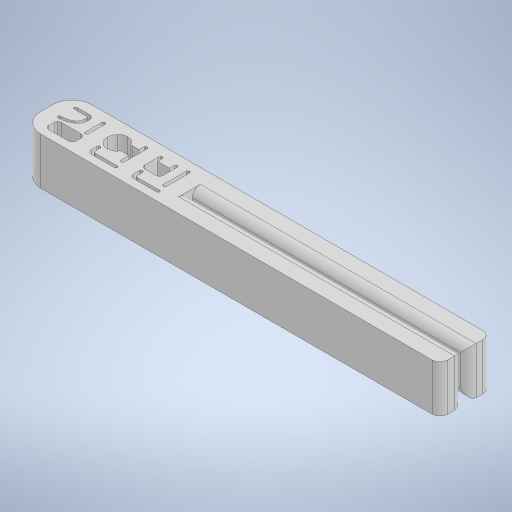
# Autodesk Inventor part: part2
Saved by Autodesk Inventor 2024 (Build 280153000, 153)
## iProperties
Created: 2023-11-09
Part Number: part2
Material: 일반
Document SubType Name: Modeling
Designer: SSAFY
Density: 1 g/cm^3
Appearance: 기본값
Author: SSAFY
Autodesk Inventor part; units mm, degrees
ref_plane "YZ Plane" through (0, 0, 0) normal (1, 0, 0) x (0, 1, 0)
ref_plane "XZ Plane" through (0, 0, 0) normal (0, 1, 0) x (-1, 0, 0)
ref_plane "XY Plane" through (0, 0, 0) normal (0, 0, 1) x (1, 0, 0)
sketch "스케치1" plane through (0, 0, 0) normal (0, 0, 1) x (1, 0, 0)
  point P0 (0, 0)
sketch "스케치2" plane through (0, 0, 0) normal (0, 1, 0) x (-1, 0, 0)
  line L0 (-38.5, 6.5) -> (38.5, 6.5)
  line L1 (38.5, 6.5) -> (38.5, -6.5)
  line L2 (38.5, -6.5) -> (-38.5, -6.5)
  line L3 (-38.5, -6.5) -> (-38.5, 6.5)
  line L4 (-38.5, 6.5) -> (38.5, -6.5) construction
  line L5 (38.5, 6.5) -> (-38.5, -6.5) construction
  line L6 (-32, 0.75) -> (32, 0.75)
  line L7 (32, 0.75) -> (32, -0.75)
  line L8 (32, -0.75) -> (-32, -0.75)
  line L9 (-32, -0.75) -> (-32, 0.75)
  line L10 (-32, 0.75) -> (32, -0.75) construction
  line L11 (32, 0.75) -> (-32, -0.75) construction
  line L12 (-32, 0.75) -> (-38.5, 0.75)
  line L13 (-38.5, 0.75) -> (-38.5, -0.75)
  line L14 (-38.5, -0.75) -> (-32, -0.75)
  line L15 (-32, -0.75) -> (-32, 0.75)
  point P0 (0, 0)
  point P1 (-32, -0.5)
  dimension "d0" = 77
  dimension "d1" = 13
  dimension "d2" = 64
  dimension "d3" = 1.5
  constraints: 32 end point, 6 parallel, 4 midpoint, 3 horizontal, 3 perpendicular, 1 point on line
  measures "d0" distance of L1.end L2.end
  measures "d1" distance of L2.end L0.start
  measures "d2" distance of L7.end L8.end
  measures "d3" distance of L8.end L6.start
extrude "돌출1" add sketch "스케치2" along normal mid plane 12 contours L0 L1 L2 L3 L14 L8 L7 L6 L12
sketch "스케치5" plane through (-38.5, -6, 6.5) normal (-1, 0, 0) x (0, 0, 1)
  line L0 (-13, 12) -> (0, 12)
  line L1 (0, 12) -> (0, 0)
  line L2 (0, 0) -> (-13, 0)
  line L3 (-13, 0) -> (-13, 12)
  point P0 (-6.5, 6)
  constraints: 8 end point, 2 parallel, 1 horizontal, 1 perpendicular
extrude "돌출3" add sketch "스케치5" along normal blind 30
sketch "스케치7" plane through (0, 6, 0) normal (0, 1, 0) x (1, 0, 0)
  line L0 (-67.5541, 5.3583) -> (-32.9181, 5.3583) construction
  line L1 (-32.9181, 5.3583) -> (-32.9181, -5.6155) construction
  line L2 (-32.9181, -5.6155) -> (-67.5541, -5.6155) construction
  line L3 (-67.5541, -5.6155) -> (-67.5541, 5.3583) construction
  line L4 (-58.4922, -1.2761) -> (-63.4387, -1.2761)
  spline S0 degree 2 poles (-63.4387, -1.2761) (-63.8795, -1.2761) (-64.1388, -1.5289) knots 0 0 0 1 1 1
  spline S1 degree 2 poles (-64.1388, -1.5289) (-64.4046, -1.7818) (-64.4046, -2.1578) knots 0 0 0 1 1 1
  line L5 (-64.4046, -2.1578) -> (-64.4046, -3.5451)
  spline S2 degree 2 poles (-64.4046, -3.5451) (-64.4046, -4.0119) (-64.1518, -4.2583) knots 0 0 0 1 1 1
  spline S3 degree 2 poles (-64.1518, -4.2583) (-63.8795, -4.5176) (-63.3025, -4.5176) knots 0 0 0 1 1 1
  line L6 (-63.3025, -4.5176) -> (-58.4468, -4.5176)
  spline S4 degree 2 poles (-58.4468, -4.5176) (-57.9865, -4.5176) (-57.6753, -4.1286) knots 0 0 0 1 1 1
  spline S5 degree 2 poles (-57.6753, -4.1286) (-57.4225, -4.0508) (-57.4225, -3.597) knots 0 0 0 1 1 1
  line L7 (-57.4225, -3.597) -> (-57.4225, -2.1189)
  spline S6 degree 2 poles (-57.4225, -2.1189) (-57.4225, -1.7364) (-57.6753, -1.5289) knots 0 0 0 1 1 1
  spline S7 degree 2 poles (-57.6753, -1.5289) (-58.0124, -1.2761) (-58.4922, -1.2761) knots 0 0 0 1 1 1
  line L8 (-58.2782, -2.2745) -> (-58.2782, -3.5322)
  spline S8 degree 2 poles (-58.2782, -3.5322) (-58.2782, -3.6618) (-58.3301, -3.7007) knots 0 0 0 1 1 1
  spline S9 degree 2 poles (-58.3301, -3.7007) (-58.4273, -3.7656) (-58.6283, -3.7656) knots 0 0 0 1 1 1
  line L9 (-58.6283, -3.7656) -> (-63.1858, -3.7656)
  spline S10 degree 2 poles (-63.1858, -3.7656) (-63.4192, -3.7656) (-63.497, -3.7007) knots 0 0 0 1 1 1
  spline S11 degree 2 poles (-63.497, -3.7007) (-63.5489, -3.6553) (-63.5489, -3.4868) knots 0 0 0 1 1 1
  line L10 (-63.5489, -3.4868) -> (-63.5489, -2.3004)
  spline S12 degree 2 poles (-63.5489, -2.3004) (-63.5489, -2.1448) (-63.4841, -2.08) knots 0 0 0 1 1 1
  spline S13 degree 2 poles (-63.4841, -2.08) (-63.4257, -2.0281) (-63.2183, -2.0281) knots 0 0 0 1 1 1
  line L11 (-63.2183, -2.0281) -> (-58.6413, -2.0281)
  spline S14 degree 2 poles (-58.6413, -2.0281) (-58.4273, -2.0281) (-58.3301, -2.0929) knots 0 0 0 1 1 1
  spline S15 degree 2 poles (-58.3301, -2.0929) (-58.2782, -2.1318) (-58.2782, -2.2745) knots 0 0 0 1 1 1
  line L12 (-61.5262, 4.0075) -> (-64.7482, 4.0075)
  spline S16 degree 2 poles (-64.7482, 4.0075) (-65.1567, 4.0075) (-65.1437, 3.638) knots 0 0 0 1 1 1
  spline S17 degree 2 poles (-65.1437, 3.638) (-65.1437, 3.2555) (-64.7418, 3.2555) knots 0 0 0 1 1 1
  line L13 (-64.7418, 3.2555) -> (-61.591, 3.2555)
  spline S18 degree 2 poles (-61.591, 3.2555) (-61.4095, 3.2555) (-61.3252, 3.1842) knots 0 0 0 1 1 1
  spline S19 degree 2 poles (-61.3252, 3.1842) (-61.215, 3.0999) (-61.215, 2.9314) knots 0 0 0 1 1 1
  line L14 (-61.215, 2.9314) -> (-61.215, 2.4711)
  spline S20 degree 2 poles (-61.215, 2.4711) (-61.215, 1.3366) (-62.0319, 0.7272) knots 0 0 0 1 1 1
  spline S21 degree 2 poles (-62.0319, 0.7272) (-63.0886, 0.0789) (-64.8455, 0.0075) knots 0 0 0 1 1 1
  spline S22 degree 2 poles (-64.8455, 0.0075) (-65.0918, 0.0075) (-65.215, -0.1156) knots 0 0 0 1 1 1
  spline S23 degree 2 poles (-65.215, -0.1156) (-65.3187, -0.2258) (-65.3187, -0.3814) knots 0 0 0 1 1 1
  spline S24 degree 2 poles (-65.3187, -0.3814) (-65.3187, -0.5435) (-65.1826, -0.6472) knots 0 0 0 1 1 1
  spline S25 degree 2 poles (-65.1826, -0.6472) (-65.0594, -0.7445) (-64.8585, -0.7445) knots 0 0 0 1 1 1
  spline S26 degree 2 poles (-64.8585, -0.7445) (-62.7515, -0.6472) (-61.5781, 0.202) knots 0 0 0 1 1 1
  spline S27 degree 2 poles (-61.5781, 0.202) (-60.3917, 1.0578) (-60.3917, 2.4646) knots 0 0 0 1 1 1
  line L15 (-60.3917, 2.4646) -> (-60.3917, 3.0221)
  spline S28 degree 2 poles (-60.3917, 3.0221) (-60.3917, 3.463) (-60.7353, 3.7482) knots 0 0 0 1 1 1
  spline S29 degree 2 poles (-60.7353, 3.7482) (-61.04, 4.0075) (-61.5262, 4.0075) knots 0 0 0 1 1 1
  line L16 (-57.4225, -0.3296) -> (-57.4225, 3.8714)
  spline S30 degree 2 poles (-57.4225, 3.8714) (-57.4225, 4.0594) (-57.5716, 4.1631) knots 0 0 0 1 1 1
  spline S31 degree 2 poles (-57.5716, 4.1631) (-57.6818, 4.2604) (-57.8504, 4.2604) knots 0 0 0 1 1 1
  spline S32 degree 2 poles (-57.8504, 4.2604) (-58.0319, 4.2604) (-58.1486, 4.1631) knots 0 0 0 1 1 1
  spline S33 degree 2 poles (-58.1486, 4.1631) (-58.2782, 4.04) (-58.2782, 3.8649) knots 0 0 0 1 1 1
  line L17 (-58.2782, 3.8649) -> (-58.2782, -0.3296)
  spline S34 degree 2 poles (-58.2782, -0.3296) (-58.2782, -0.5241) (-58.1551, -0.6472) knots 0 0 0 1 1 1
  spline S35 degree 2 poles (-58.1551, -0.6472) (-58.0384, -0.7639) (-57.8504, -0.7639) knots 0 0 0 1 1 1
  spline S36 degree 2 poles (-57.8504, -0.7639) (-57.6753, -0.7639) (-57.5457, -0.6343) knots 0 0 0 1 1 1
  spline S37 degree 2 poles (-57.5457, -0.6343) (-57.4225, -0.5241) (-57.4225, -0.3296) knots 0 0 0 1 1 1
  spline S38 degree 2 poles (-51.7628, 3.9881) (-52.9622, 3.9881) (-53.6688, 3.1583) knots 0 0 0 1 1 1
  spline S39 degree 2 poles (-53.6688, 3.1583) (-54.2977, 2.4257) (-54.2977, 1.356) knots 0 0 0 1 1 1
  spline S40 degree 2 poles (-54.2977, 1.356) (-54.2977, 0.2928) (-53.6948, -0.3425) knots 0 0 0 1 1 1
  spline S41 degree 2 poles (-53.6948, -0.3425) (-52.9622, -1.2826) (-51.7628, -1.2826) knots 0 0 0 1 1 1
  spline S42 degree 2 poles (-51.7628, -1.2826) (-50.5829, -1.2826) (-49.8893, -0.4527) knots 0 0 0 1 1 1
  spline S43 degree 2 poles (-49.8893, -0.4527) (-49.2604, 0.2863) (-49.2604, 1.356) knots 0 0 0 1 1 1
  spline S44 degree 2 poles (-49.2604, 1.356) (-49.2604, 2.4257) (-49.8893, 3.1583) knots 0 0 0 1 1 1
  spline S45 degree 2 poles (-49.8893, 3.1583) (-50.5829, 3.9881) (-51.7628, 3.9881) knots 0 0 0 1 1 1
  spline S46 degree 2 poles (-51.7628, 3.2361) (-50.9654, 3.2361) (-50.5181, 2.6656) knots 0 0 0 1 1 1
  spline S47 degree 2 poles (-50.5181, 2.6656) (-50.0902, 2.134) (-50.0902, 1.356) knots 0 0 0 1 1 1
  spline S48 degree 2 poles (-50.0902, 1.356) (-50.0902, 0.5716) (-50.5246, 0.0335) knots 0 0 0 1 1 1
  spline S49 degree 2 poles (-50.5246, 0.0335) (-50.9654, -0.5305) (-51.7628, -0.5305) knots 0 0 0 1 1 1
  spline S50 degree 2 poles (-51.7628, -0.5305) (-52.5797, -0.5305) (-53.0335, 0.0529) knots 0 0 0 1 1 1
  spline S51 degree 2 poles (-53.0335, 0.0529) (-53.4419, 0.5651) (-53.4419, 1.356) knots 0 0 0 1 1 1
  spline S52 degree 2 poles (-53.4419, 1.356) (-53.4419, 2.1404) (-53.0335, 2.6591) knots 0 0 0 1 1 1
  spline S53 degree 2 poles (-53.0335, 2.6591) (-52.5732, 3.2361) (-51.7628, 3.2361) knots 0 0 0 1 1 1
  line L18 (-46.6283, -1.9438) -> (-46.6283, 3.8714)
  spline S54 degree 2 poles (-46.6283, 3.8714) (-46.6283, 4.0594) (-46.7709, 4.1567) knots 0 0 0 1 1 1
  spline S55 degree 2 poles (-46.7709, 4.1567) (-46.8876, 4.2604) (-47.0562, 4.2604) knots 0 0 0 1 1 1
  spline S56 degree 2 poles (-47.0562, 4.2604) (-47.2377, 4.2604) (-47.3544, 4.1631) knots 0 0 0 1 1 1
  spline S57 degree 2 poles (-47.3544, 4.1631) (-47.4841, 4.0464) (-47.4841, 3.8649) knots 0 0 0 1 1 1
  line L19 (-47.4841, 3.8649) -> (-47.4841, 2.6202)
  line L20 (-47.4841, 2.6202) -> (-49.1696, 2.6202)
  spline S58 degree 2 poles (-49.1696, 2.6202) (-49.3771, 2.6202) (-49.4938, 2.5165) knots 0 0 0 1 1 1
  spline S59 degree 2 poles (-49.4938, 2.5165) (-49.5975, 2.3998) (-49.5975, 2.2377) knots 0 0 0 1 1 1
  spline S60 degree 2 poles (-49.5975, 2.2377) (-49.5846, 2.0951) (-49.4743, 1.9849) knots 0 0 0 1 1 1
  spline S61 degree 2 poles (-49.4743, 1.9849) (-49.3252, 1.8682) (-49.1178, 1.8682) knots 0 0 0 1 1 1
  line L21 (-49.1178, 1.8682) -> (-47.4841, 1.8682)
  line L22 (-47.4841, 1.8682) -> (-47.4841, 0.7012)
  line L23 (-47.4841, 0.7012) -> (-49.1502, 0.7012)
  spline S62 degree 2 poles (-49.1502, 0.7012) (-49.3447, 0.7012) (-49.4808, 0.5975) knots 0 0 0 1 1 1
  spline S63 degree 2 poles (-49.4808, 0.5975) (-49.5846, 0.4938) (-49.5846, 0.3382) knots 0 0 0 1 1 1
  spline S64 degree 2 poles (-49.5846, 0.3382) (-49.5846, 0.1761) (-49.4614, 0.0724) knots 0 0 0 1 1 1
  spline S65 degree 2 poles (-49.4614, 0.0724) (-49.3382, -0.0378) (-49.1372, -0.0378) knots 0 0 0 1 1 1
  line L24 (-49.1372, -0.0378) -> (-47.4841, -0.0378)
  line L25 (-47.4841, -0.0378) -> (-47.4841, -1.9438)
  spline S66 degree 2 poles (-47.4841, -1.9438) (-47.4841, -2.1513) (-47.3609, -2.2745) knots 0 0 0 1 1 1
  spline S67 degree 2 poles (-47.3609, -2.2745) (-47.2442, -2.3912) (-47.0562, -2.3912) knots 0 0 0 1 1 1
  spline S68 degree 2 poles (-47.0562, -2.3912) (-46.8811, -2.3912) (-46.7515, -2.2615) knots 0 0 0 1 1 1
  spline S69 degree 2 poles (-46.7515, -2.2615) (-46.6283, -2.1513) (-46.6283, -1.9438) knots 0 0 0 1 1 1
  spline S70 degree 2 poles (-52.7677, -2.067) (-52.7677, -1.8531) (-52.8909, -1.7429) knots 0 0 0 1 1 1
  spline S71 degree 2 poles (-52.8909, -1.7429) (-53.0205, -1.6132) (-53.1956, -1.6132) knots 0 0 0 1 1 1
  spline S72 degree 2 poles (-53.1956, -1.6132) (-53.3836, -1.6132) (-53.5003, -1.7299) knots 0 0 0 1 1 1
  spline S73 degree 2 poles (-53.5003, -1.7299) (-53.6234, -1.8531) (-53.6234, -2.067) knots 0 0 0 1 1 1
  line L26 (-53.6234, -2.067) -> (-53.6234, -3.4673)
  spline S74 degree 2 poles (-53.6234, -3.4673) (-53.6234, -3.986) (-53.2799, -4.2712) knots 0 0 0 1 1 1
  spline S75 degree 2 poles (-53.2799, -4.2712) (-52.9881, -4.5176) (-52.4695, -4.5176) knots 0 0 0 1 1 1
  line L27 (-52.4695, -4.5176) -> (-46.6867, -4.5176)
  spline S76 degree 2 poles (-46.6867, -4.5176) (-46.3106, -4.5176) (-46.3106, -4.1351) knots 0 0 0 1 1 1
  spline S77 degree 2 poles (-46.3106, -4.1351) (-46.3106, -3.7656) (-46.6867, -3.7656) knots 0 0 0 1 1 1
  line L28 (-46.6867, -3.7656) -> (-52.3593, -3.7656)
  spline S78 degree 2 poles (-52.3593, -3.7656) (-52.6251, -3.7656) (-52.6834, -3.7137) knots 0 0 0 1 1 1
  spline S79 degree 2 poles (-52.6834, -3.7137) (-52.7677, -3.6294) (-52.7677, -3.3831) knots 0 0 0 1 1 1
  line L29 (-52.7677, -3.3831) -> (-52.7677, -2.067)
  line L30 (-39.5165, 3.5991) -> (-39.5165, 2.3868)
  line L31 (-39.5165, 2.3868) -> (-42.5311, 2.3868)
  line L32 (-42.5311, 2.3868) -> (-42.5311, 3.5473)
  spline S80 degree 2 poles (-42.5311, 3.5473) (-42.5311, 3.7612) (-42.6542, 3.8714) knots 0 0 0 1 1 1
  spline S81 degree 2 poles (-42.6542, 3.8714) (-42.7839, 4.0011) (-42.9589, 4.0011) knots 0 0 0 1 1 1
  spline S82 degree 2 poles (-42.9589, 4.0011) (-43.134, 4.0011) (-43.2377, 3.8844) knots 0 0 0 1 1 1
  spline S83 degree 2 poles (-43.2377, 3.8844) (-43.3739, 3.7482) (-43.3739, 3.5408) knots 0 0 0 1 1 1
  line L33 (-43.3739, 3.5408) -> (-43.3739, -0.0443)
  spline S84 degree 2 poles (-43.3739, -0.0443) (-43.3739, -0.4852) (-43.1081, -0.7186) knots 0 0 0 1 1 1
  spline S85 degree 2 poles (-43.1081, -0.7186) (-42.8098, -0.9649) (-42.3755, -0.9649) knots 0 0 0 1 1 1
  line L34 (-42.3755, -0.9649) -> (-39.7304, -0.9649)
  spline S86 degree 2 poles (-39.7304, -0.9649) (-39.2766, -0.9649) (-38.9978, -0.7121) knots 0 0 0 1 1 1
  spline S87 degree 2 poles (-38.9978, -0.7121) (-38.6931, -0.4527) (-38.6931, -0.0443) knots 0 0 0 1 1 1
  line L35 (-38.6931, -0.0443) -> (-38.6931, 3.5926)
  spline S88 degree 2 poles (-38.6931, 3.5926) (-38.6931, 4.0011) (-39.1081, 4.0011) knots 0 0 0 1 1 1
  spline S89 degree 2 poles (-39.1081, 4.0011) (-39.5165, 4.0011) (-39.5165, 3.5991) knots 0 0 0 1 1 1
  spline S90 degree 2 poles (-41.9735, -2.067) (-41.9735, -1.8531) (-42.0967, -1.7429) knots 0 0 0 1 1 1
  spline S91 degree 2 poles (-42.0967, -1.7429) (-42.2264, -1.6132) (-42.4014, -1.6132) knots 0 0 0 1 1 1
  spline S92 degree 2 poles (-42.4014, -1.6132) (-42.5894, -1.6132) (-42.7061, -1.7299) knots 0 0 0 1 1 1
  spline S93 degree 2 poles (-42.7061, -1.7299) (-42.8293, -1.8531) (-42.8293, -2.067) knots 0 0 0 1 1 1
  line L36 (-42.8293, -2.067) -> (-42.8293, -3.4673)
  spline S94 degree 2 poles (-42.8293, -3.4673) (-42.8293, -3.986) (-42.4857, -4.2712) knots 0 0 0 1 1 1
  spline S95 degree 2 poles (-42.4857, -4.2712) (-42.194, -4.5176) (-41.6753, -4.5176) knots 0 0 0 1 1 1
  line L37 (-41.6753, -4.5176) -> (-35.8925, -4.5176)
  spline S96 degree 2 poles (-35.8925, -4.5176) (-35.5165, -4.5176) (-35.5165, -4.1351) knots 0 0 0 1 1 1
  spline S97 degree 2 poles (-35.5165, -4.1351) (-35.5165, -3.7656) (-35.8925, -3.7656) knots 0 0 0 1 1 1
  line L38 (-35.8925, -3.7656) -> (-41.5651, -3.7656)
  spline S98 degree 2 poles (-41.5651, -3.7656) (-41.8309, -3.7656) (-41.8893, -3.7137) knots 0 0 0 1 1 1
  spline S99 degree 2 poles (-41.8893, -3.7137) (-41.9735, -3.6294) (-41.9735, -3.3831) knots 0 0 0 1 1 1
  line L39 (-41.9735, -3.3831) -> (-41.9735, -2.067)
  line L40 (-35.8341, -1.9438) -> (-35.8341, 3.8714)
  spline S100 degree 2 poles (-35.8341, 3.8714) (-35.8341, 4.0594) (-35.9768, 4.1567) knots 0 0 0 1 1 1
  spline S101 degree 2 poles (-35.9768, 4.1567) (-36.0935, 4.2604) (-36.262, 4.2604) knots 0 0 0 1 1 1
  spline S102 degree 2 poles (-36.262, 4.2604) (-36.4435, 4.2604) (-36.5602, 4.1631) knots 0 0 0 1 1 1
  spline S103 degree 2 poles (-36.5602, 4.1631) (-36.6899, 4.04) (-36.6899, 3.8649) knots 0 0 0 1 1 1
  line L41 (-36.6899, 3.8649) -> (-36.6899, -1.9438)
  spline S104 degree 2 poles (-36.6899, -1.9438) (-36.6899, -2.1513) (-36.5667, -2.2745) knots 0 0 0 1 1 1
  spline S105 degree 2 poles (-36.5667, -2.2745) (-36.45, -2.3912) (-36.262, -2.3912) knots 0 0 0 1 1 1
  spline S106 degree 2 poles (-36.262, -2.3912) (-36.087, -2.3912) (-35.9573, -2.2615) knots 0 0 0 1 1 1
  spline S107 degree 2 poles (-35.9573, -2.2615) (-35.8341, -2.1513) (-35.8341, -1.9438) knots 0 0 0 1 1 1
  line L42 (-39.5165, 1.6348) -> (-39.5165, 0.0853)
  spline S108 degree 2 poles (-39.5165, 0.0853) (-39.5165, -0.0767) (-39.6137, -0.1416) knots 0 0 0 1 1 1
  spline S109 degree 2 poles (-39.6137, -0.1416) (-39.698, -0.2129) (-39.9119, -0.2129) knots 0 0 0 1 1 1
  line L43 (-39.9119, -0.2129) -> (-42.2069, -0.2129)
  spline S110 degree 2 poles (-42.2069, -0.2129) (-42.4079, -0.2129) (-42.4598, -0.161) knots 0 0 0 1 1 1
  spline S111 degree 2 poles (-42.4598, -0.161) (-42.5311, -0.1027) (-42.5311, 0.0853) knots 0 0 0 1 1 1
  line L44 (-42.5311, 0.0853) -> (-42.5311, 1.6348)
  line L45 (-42.5311, 1.6348) -> (-39.5165, 1.6348)
  point P0 (0, 0)
  constraints: 2 other
emboss "엠보싱3" sketch "스케치7" operation cut depth 15 direction (0, -1, 0) contours S7 S6 L7 S5 S4 L6 S3 S2 L5 S1 S0 L4 | S29 S28 L15 S27 S26 S25 S24 S23 S22 S21 S20 L14 S19 S18 L13 S17 S16 L12 | S37 S36 S35 S34 L17 S33 S32 S31 S30 L16 | S45 S44 S58 S59 S60 S61 S43 S62 S63 S64 S42 S41 S40 S39 S38 | S58 L20 L19 S57 S56 S55 S54 L18 S69 S68 S67 S66 L25 L24 S65 S64 S43 S62 L23 L22 L21 S61 S44 | S44 S61 S60 S59 S58 | S43 S64 S63 S62 | L29 S79 S78 L28 S77 S76 L27 S75 S74 L26 S73 S72 S71 S70 | S89 S88 L35 S87 S86 L34 S85 S84 L33 S83 S82 S81 S80 L32 L31 L30 | L39 S99 S98 L38 S97 S96 L37 S95 S94 L36 S93 S92 S91 S90 | S107 S106 S105 S104 L41 S103 S102 S101 S100 L40
sketch "스케치8" plane through (0, 6, 0) normal (0, 1, 0) x (1, 0, 0)
  spline S0 degree 6 poles (-63.497, -3.7007) (-63.4703, -3.723) (-63.4326, -3.7406) (-63.3844, -3.7534) (-63.3266, -3.7616) (-63.2601, -3.7656) (-63.1858, -3.7656) knots 0 0 0 0 0 0 0 1 1 1 1 1 1 1 projected
  line L0 (-63.1858, -3.7656) -> (-58.6283, -3.7656) projected
  spline S1 degree 5 poles (-58.6283, -3.7656) (-58.5502, -3.7656) (-58.4804, -3.7594) (-58.42, -3.7467) (-58.3698, -3.7272) (-58.3301, -3.7007) knots 0 0 0 0 0 0 1 1 1 1 1 1 projected
  spline S2 degree 5 poles (-58.3301, -3.7007) (-58.3092, -3.685) (-58.2935, -3.6601) (-58.2833, -3.6261) (-58.2782, -3.5832) (-58.2782, -3.5322) knots 0 0 0 0 0 0 1 1 1 1 1 1 projected
  line L1 (-58.2782, -3.5322) -> (-58.2782, -2.2745) projected
  spline S3 degree 5 poles (-58.2782, -2.2745) (-58.2782, -2.2185) (-58.2832, -2.1718) (-58.2935, -2.135) (-58.3091, -2.1087) (-58.3301, -2.0929) knots 0 0 0 0 0 0 1 1 1 1 1 1 projected
  spline S4 degree 5 poles (-58.3301, -2.0929) (-58.3699, -2.0664) (-58.4218, -2.0468) (-58.485, -2.0342) (-58.5585, -2.0281) (-58.6413, -2.0281) knots 0 0 0 0 0 0 1 1 1 1 1 1 projected
  line L2 (-58.6413, -2.0281) -> (-63.2183, -2.0281) projected
  spline S5 degree 6 poles (-63.2183, -2.0281) (-63.2847, -2.0281) (-63.3433, -2.0313) (-63.3932, -2.0379) (-63.4337, -2.0482) (-63.4641, -2.0622) (-63.4841, -2.08) knots 0 0 0 0 0 0 0 1 1 1 1 1 1 1 projected
  spline S6 degree 5 poles (-63.4841, -2.08) (-63.5103, -2.1062) (-63.5298, -2.1417) (-63.5426, -2.1862) (-63.5489, -2.2393) (-63.5489, -2.3004) knots 0 0 0 0 0 0 1 1 1 1 1 1 projected
  line L3 (-63.5489, -2.3004) -> (-63.5489, -3.4868) projected
  spline S7 degree 5 poles (-63.5489, -3.4868) (-63.5489, -3.5524) (-63.544, -3.6075) (-63.5338, -3.6511) (-63.5181, -3.6823) (-63.497, -3.7007) knots 0 0 0 0 0 0 1 1 1 1 1 1 projected
  spline S8 degree 5 poles (-51.7628, -0.5305) (-51.6946, -0.5305) (-51.6268, -0.528) (-51.5597, -0.5226) (-51.4932, -0.5143) (-51.3117, -0.4829) (-51.1986, -0.453) (-51.0897, -0.4127) (-50.9863, -0.3616) (-50.806, -0.2475) (-50.7274, -0.1872) (-50.6542, -0.1197) (-50.5866, -0.0459) (-50.5246, 0.0335) knots 0 0 0 0 0 0 0.232634 0.232634 0.232634 0.232634 0.645224 0.645224 0.645224 0.645224 1 1 1 1 1 1 projected
  spline S9 degree 6 poles (-50.5246, 0.0335) (-50.4921, 0.0738) (-50.4609, 0.115) (-50.4311, 0.1573) (-50.4027, 0.2004) (-50.3758, 0.2444) (-50.2608, 0.4477) (-50.1896, 0.6166) (-50.1381, 0.7941) (-50.1055, 0.9779) (-50.0902, 1.1658) (-50.0902, 1.356) knots 0 0 0 0 0 0 0 0.220725 0.220725 0.220725 0.220725 0.220725 1 1 1 1 1 1 1 projected
  spline S10 degree 6 poles (-50.0902, 1.356) (-50.0902, 1.5473) (-50.1058, 1.7362) (-50.1388, 1.9209) (-50.1911, 2.0991) (-50.2634, 2.2684) (-50.3786, 2.4685) (-50.404, 2.5096) (-50.4306, 2.5498) (-50.4586, 2.5893) (-50.4877, 2.6278) (-50.5181, 2.6656) knots 0 0 0 0 0 0 0 0.791229 0.791229 0.791229 0.791229 0.791229 1 1 1 1 1 1 1 projected
  spline S11 degree 5 poles (-50.5181, 2.6656) (-50.5837, 2.7492) (-50.6553, 2.8269) (-50.733, 2.8975) (-50.8165, 2.9603) (-51.0015, 3.0738) (-51.104, 3.1231) (-51.2117, 3.1619) (-51.3232, 3.1906) (-51.5012, 3.2207) (-51.5657, 3.2285) (-51.6309, 3.2336) (-51.6967, 3.2361) (-51.7628, 3.2361) knots 0 0 0 0 0 0 0.371373 0.371373 0.371373 0.371373 0.775292 0.775292 0.775292 0.775292 1 1 1 1 1 1 projected
  spline S12 degree 5 poles (-51.7628, 3.2361) (-51.8301, 3.2361) (-51.897, 3.2336) (-51.9633, 3.2285) (-52.0289, 3.2205) (-52.2101, 3.1901) (-52.3238, 3.1611) (-52.4335, 3.1218) (-52.5381, 3.0719) (-52.7273, 2.9571) (-52.8128, 2.8937) (-52.8925, 2.8222) (-52.966, 2.7437) (-53.0335, 2.6591) knots 0 0 0 0 0 0 0.224613 0.224613 0.224613 0.224613 0.628567 0.628567 0.628567 0.628567 1 1 1 1 1 1 projected
  spline S13 degree 6 poles (-53.0335, 2.6591) (-53.0501, 2.638) (-53.0663, 2.6167) (-53.0821, 2.5951) (-53.0975, 2.5732) (-53.1125, 2.551) (-53.2366, 2.3603) (-53.3232, 2.1772) (-53.3852, 1.9819) (-53.4239, 1.778) (-53.4419, 1.5685) (-53.4419, 1.356) knots 0 0 0 0 0 0 0 0.117636 0.117636 0.117636 0.117636 0.117636 1 1 1 1 1 1 1 projected
  spline S14 degree 6 poles (-53.4419, 1.356) (-53.4419, 1.2427) (-53.4369, 1.1303) (-53.4264, 1.0192) (-53.4101, 0.9098) (-53.3875, 0.8026) (-53.3314, 0.6005) (-53.2988, 0.5054) (-53.2603, 0.4129) (-53.2158, 0.3236) (-53.1656, 0.2379) (-53.0976, 0.1384) (-53.0853, 0.1209) (-53.0727, 0.1036) (-53.0599, 0.0865) (-53.0468, 0.0696) (-53.0335, 0.0529) knots 0 0 0 0 0 0 0 0.469073 0.469073 0.469073 0.469073 0.469073 0.905935 0.905935 0.905935 0.905935 0.905935 1 1 1 1 1 1 1 projected
  spline S15 degree 5 poles (-53.0335, 0.0529) (-52.9679, -0.0315) (-52.8961, -0.1099) (-52.8183, -0.1815) (-52.7345, -0.2451) (-52.5471, -0.3617) (-52.4422, -0.4129) (-52.3319, -0.4531) (-52.2175, -0.483) (-52.0343, -0.5144) (-51.9674, -0.5226) (-51.8997, -0.528) (-51.8315, -0.5305) (-51.7628, -0.5305) knots 0 0 0 0 0 0 0.366043 0.366043 0.366043 0.366043 0.77173 0.77173 0.77173 0.77173 1 1 1 1 1 1 projected
  line L4 (-49.1502, 0.7012) -> (-47.4841, 0.7012) projected
  line L5 (-47.4841, 0.7012) -> (-47.4841, 1.8682) projected
  line L6 (-47.4841, 1.8682) -> (-49.1178, 1.8682) projected
  spline S16 degree 5 poles (-49.1178, 1.8682) (-49.1574, 1.8682) (-49.1959, 1.8708) (-49.2331, 1.8762) (-49.2692, 1.8843) (-49.3039, 1.8952) knots 0 0 0 0 0 0 1 1 1 1 1 1 projected
  spline S17 degree 5 poles (-49.3039, 1.8952) (-49.3024, 1.8865) (-49.301, 1.8779) (-49.2996, 1.8693) (-49.2983, 1.8607) (-49.2819, 1.7542) (-49.271, 1.6555) (-49.2639, 1.5561) (-49.2604, 1.4562) (-49.2604, 1.356) knots 0 0 0 0 0 0 0.081208 0.081208 0.081208 0.081208 1 1 1 1 1 1 projected
  spline S18 degree 5 poles (-49.2604, 1.356) (-49.2604, 1.2574) (-49.2637, 1.159) (-49.2706, 1.0611) (-49.2812, 0.9639) (-49.3016, 0.8287) (-49.308, 0.79) (-49.3151, 0.7515) (-49.3229, 0.7131) (-49.3313, 0.6749) knots 0 0 0 0 0 0 0.712767 0.712767 0.712767 0.712767 1 1 1 1 1 1 projected
  spline S19 degree 5 poles (-49.3313, 0.6749) (-49.2978, 0.6855) (-49.263, 0.6934) (-49.2267, 0.6986) (-49.1891, 0.7012) (-49.1502, 0.7012) knots 0 0 0 0 0 0 1 1 1 1 1 1 projected
  line L7 (-42.2069, -0.2129) -> (-39.9119, -0.2129) projected
  spline S20 degree 6 poles (-39.9119, -0.2129) (-39.8432, -0.2129) (-39.7811, -0.2085) (-39.7266, -0.1993) (-39.6802, -0.1852) (-39.6425, -0.1659) (-39.6137, -0.1416) knots 0 0 0 0 0 0 0 1 1 1 1 1 1 1 projected
  spline S21 degree 5 poles (-39.6137, -0.1416) (-39.6072, -0.1372) (-39.6009, -0.1326) (-39.5949, -0.1277) (-39.5892, -0.1225) (-39.5566, -0.0898) (-39.5363, -0.0557) (-39.523, -0.0149) (-39.5165, 0.0323) (-39.5165, 0.0853) knots 0 0 0 0 0 0 0.1669 0.1669 0.1669 0.1669 1 1 1 1 1 1 projected
  line L8 (-39.5165, 0.0853) -> (-39.5165, 1.6348) projected
  line L9 (-39.5165, 1.6348) -> (-42.5311, 1.6348) projected
  line L10 (-42.5311, 1.6348) -> (-42.5311, 0.0853) projected
  spline S22 degree 5 poles (-42.5311, 0.0853) (-42.5311, 0.0124) (-42.5244, -0.0498) (-42.5104, -0.1001) (-42.4888, -0.1372) (-42.4598, -0.161) knots 0 0 0 0 0 0 1 1 1 1 1 1 projected
  spline S23 degree 6 poles (-42.4598, -0.161) (-42.442, -0.1787) (-42.4139, -0.1928) (-42.3757, -0.203) (-42.3279, -0.2097) (-42.2713, -0.2129) (-42.2069, -0.2129) knots 0 0 0 0 0 0 0 1 1 1 1 1 1 1 projected
  point P0 (0, 0)
  constraints: 24 other
extrude "돌출4" cut sketch "스케치8" against normal through all
fillet "모깎기3" radius 2 8 edges at (3.25, 6, 0.75) (3.25, 6, -0.75) (3.25, -6, 0.75) (3.25, -6, -0.75) (38.5, 0, 0.75) (38.5, 0, 6.5) (38.5, 0, -0.75) (38.5, 0, -6.5)
fillet "모깎기4" radius 5 2 edges at (-68.5, 0, 6.5) (-68.5, 0, -6.5)
sketch "스케치6" plane through (38.5, -6, 6.5) normal (0, 0, 1) x (1, 0, 0)
  line L0 (-106.7099, 11.874) -> (-75.4105, 11.874) construction
  line L1 (-75.4105, 11.874) -> (-75.4105, 0.0773) construction
  line L2 (-75.4105, 0.0773) -> (-106.7099, 0.0773) construction
  line L3 (-106.7099, 0.0773) -> (-106.7099, 11.874) construction
  point P0 (-38.5, 6)
  constraints: 2 other
